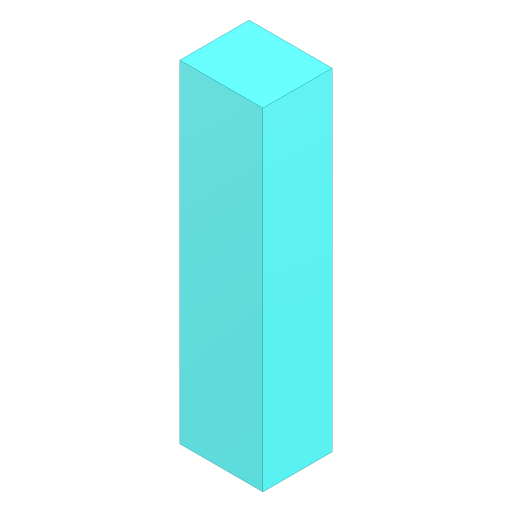
# Autodesk Inventor part: trimmed_block
Saved by Autodesk Inventor 2024 (Build 280153000, 153)
## iProperties
Created: 2023-08-28
Part Number: trimmed_block
Material: 一般
Document SubType Name: Modeling
Designer: admin
Density: 1 g/cm^3
Appearance: 平滑 - 紅色
Author: admin
Autodesk Inventor part; units mm, degrees
ref_plane "YZ Plane" through (0, 0, 0) normal (1, 0, 0) x (0, 1, 0)
ref_plane "XZ Plane" through (0, 0, 0) normal (0, 1, 0) x (-1, 0, 0)
ref_plane "XY Plane" through (0, 0, 0) normal (0, 0, 1) x (1, 0, 0)
sketch "草圖4" plane through (0, 0, 0) normal (0, 1, 0) x (-1, 0, 0)
  line L0 (12, 10) -> (-12, 10)
  line L1 (-12, 10) -> (-12, -10)
  line L2 (-12, -10) -> (12, -10)
  line L3 (12, -10) -> (12, 10)
  line L4 (12, 10) -> (-12, -10) construction
  line L5 (-12, 10) -> (12, -10) construction
  point P0 (0, 0)
  point P1 (0, 0)
  dimension "d23" = 20
  dimension "d24" = 24
  constraints: 12 end point, 2 midpoint, 2 parallel, 1 coincident, 1 horizontal, 1 perpendicular
  measures "d23" distance of L2.end L0.start
  measures "d24" distance of L1.end L2.end
extrude "擠出4" add sketch "草圖4" along normal blind 96
equation "\"width\" = 80 * ratio"
equation "\"height\" = 20 * ratio"
equation "\"length\" = width"
equation "\"leg_length\" = ratio"
equation "\"ratio\" = 1.2"
equation "\"thickness\" = 5 * ratio"
